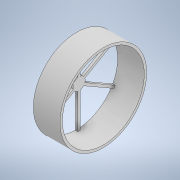
# Autodesk Inventor part: SuportMotor
Saved by Autodesk Inventor 2020.3 (Build 243373000, 373)
## iProperties
Created: 2021-03-13
Part Number: SuportMotor
Material: Generic
Document SubType Name: Modeling
Designer: alexo
Density: 1 g/cm^3
Appearance: Default
Author: alexo
Autodesk Inventor part; units mm, degrees
ref_plane "YZ Plane" through (0, 0, 0) normal (1, 0, 0) x (0, 1, 0)
ref_plane "XZ Plane" through (0, 0, 0) normal (0, 1, 0) x (-1, 0, 0)
ref_plane "XY Plane" through (0, 0, 0) normal (0, 0, 1) x (1, 0, 0)
sketch "Sketch1" plane through (0, 0, 0) normal (1, 0, 0) x (0, 1, 0)
  arc A0 (35.4672, -57.431) -> (67.4704, -2) centre (0, 0) ccw
  circle A1 centre (0, 0) radius 71.5
  arc A2 (3.1669, 9.4853) -> (-3.1669, 9.4853) centre (0, 0) ccw
  line L0 (10, 0) -> (67.5, 0) construction
  line L1 (9.798, 2) -> (67.4704, 2)
  line L2 (9.798, -2) -> (67.4704, -2)
  line L3 (3.1669, 9.4853) -> (32.0031, 59.431)
  line L4 (6.631, 7.4853) -> (35.4672, 57.431)
  line L5 (-6.631, 7.4853) -> (-35.4672, 57.431)
  line L6 (-3.1669, 9.4853) -> (-32.0031, 59.431)
  line L7 (-9.798, -2) -> (-67.4704, -2)
  line L8 (-9.798, 2) -> (-67.4704, 2)
  line L9 (-3.1669, -9.4853) -> (-32.0031, -59.431)
  line L10 (-6.631, -7.4853) -> (-35.4672, -57.431)
  line L11 (6.631, -7.4853) -> (35.4672, -57.431)
  line L12 (3.1669, -9.4853) -> (32.0031, -59.431)
  arc A3 (6.631, 7.4853) -> (3.1669, 9.4853) centre (0, 0) ccw
  arc A4 (-6.631, 7.4853) -> (-9.798, 2) centre (0, 0) ccw
  arc A5 (-3.1669, 9.4853) -> (-6.631, 7.4853) centre (0, 0) ccw
  arc A6 (-9.798, 2) -> (-9.798, -2) centre (0, 0) ccw
  arc A7 (-9.798, -2) -> (-6.631, -7.4853) centre (0, 0) ccw
  arc A8 (-6.631, -7.4853) -> (-3.1669, -9.4853) centre (0, 0) ccw
  arc A9 (-3.1669, -9.4853) -> (3.1669, -9.4853) centre (0, 0) ccw
  arc A10 (3.1669, -9.4853) -> (6.631, -7.4853) centre (0, 0) ccw
  arc A11 (6.631, -7.4853) -> (6.631, 7.4853) centre (0, 0) ccw
  arc A12 (32.0031, -59.431) -> (35.4672, -57.431) centre (0, 0) ccw
  arc A13 (67.4704, -2) -> (67.4704, 2) centre (0, 0) ccw construction
  arc A14 (35.4672, 57.431) -> (32.0031, 59.431) centre (0, 0) ccw construction
  arc A15 (32.0031, 59.431) -> (-32.0031, 59.431) centre (0, 0) ccw
  arc A16 (-32.0031, 59.431) -> (-35.4672, 57.431) centre (0, 0) ccw construction
  arc A17 (-35.4672, 57.431) -> (-67.4704, 2) centre (0, 0) ccw
  arc A18 (-67.4704, 2) -> (-67.4704, -2) centre (0, 0) ccw construction
  arc A19 (-67.4704, -2) -> (-35.4672, -57.431) centre (0, 0) ccw
  arc A20 (-35.4672, -57.431) -> (-32.0031, -59.431) centre (0, 0) ccw construction
  arc A21 (-32.0031, -59.431) -> (32.0031, -59.431) centre (0, 0) ccw
  arc A22 (67.4704, 2) -> (35.4672, 57.431) centre (0, 0) ccw
  dimension "d0" = 135
  dimension "d1" = 4
  dimension "d2" = 20
  dimension "d3" = 2
  dimension "d4" = 2
  dimension "d7" = 360
  constraints: 74 point on circle, 26 end point, 23 centre point, 9 line through centre, 2 coincident, 2 parallel, 1 horizontal, 37 other
  measures "d0" diameter of A0
  measures "d1" radial gap between concentric circles of A0 A1
  measures "d2" diameter of A2
  measures "d3" distance between parallel lines of L0 L1
  measures "d4" distance between parallel lines of L0 L2
extrude "Extrusion1" add sketch "Sketch1" along normal blind 4 contours A12 L12 A10 L11 | A10 A9 A8 A7 A6 A4 A5 A2 A3 A11 | A1
sketch "Sketch2" plane through (4, 0, 0) normal (1, 0, 0) x (0, 0, -1)
  circle A0 centre (0, 0) radius 71.5 projected
  line L0 (-59.431, 32.0031) -> (-9.4853, 3.1669) projected
  circle A1 centre (0, 0) radius 67.5
  constraints: 1 coincident, 3 other
extrude "Extrusion2" add sketch "Sketch2" along normal blind 40
body "Solid1"
